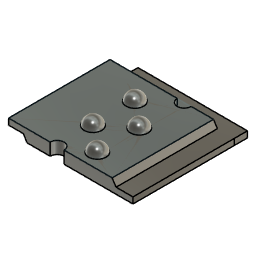
Rivets-Double riveted zig-zag lap joint (Autodesk Fusion 360 design; units mm, degrees)
Autodesk Fusion 360 part; units mm, degrees
sketch "Sketch1" plane through (0, 0, 0) normal (0, 1, 0) x (1, 0, 0)
  line L0 (0, 0) -> (-29, 0)
  line L1 (0, 0) -> (29, 0)
  line L2 (29, 0) -> (29, -7)
  line L3 (29, 0) -> (29, 7)
  line L4 (-29, 0) -> (-29, -7)
  line L5 (-29, 0) -> (-29, 7)
  line L6 (29, 0) -> (53, 0)
  line L7 (-29, 0) -> (-53, 0)
  line L8 (-29, -7) -> (-70, -7)
  line L9 (-70, -7) -> (48.4788, -7)
  line L10 (-29, 7) -> (72.2751, 7)
  line L11 (53, 0) -> (48.4788, -7)
  line L12 (-53, 0) -> (-70, 0)
  line L13 (53, 0) -> (72.2751, 0)
  line L14 (72.2751, 0) -> (72.2751, 7)
  line L15 (-29, -7) -> (-53, -7)
  line L16 (-53, 0) -> (-49.003, 7)
  line L17 (0, 7) -> (-49.003, 7)
  line L18 (-70, -7) -> (-70, 0)
  dimension "d1" = 29
  dimension "d2" = 29
  dimension "d3" = 7
  dimension "d4" = 7
  dimension "d5" = 7
  dimension "d6" = 7
  dimension "d8" = 24
  dimension "d9" = 24
  dimension "d15" = 24
  dimension "d16" = 7
  constraint coincident L0.start L1.start
  constraint horizontal L0
  constraint parallel L0 L1
  constraint perpendicular L1 L2
  constraint perpendicular L1 L3
  constraint perpendicular L0 L4
  constraint perpendicular L0 L5
  constraint perpendicular L2 L6
  constraint perpendicular L5 L7
  constraint perpendicular L4 L8
  constraint perpendicular L2 L9
  constraint perpendicular L3 L10
  constraint parallel L7 L12
  constraint parallel L10 L13
  constraint perpendicular L10 L14
  constraint perpendicular L4 L15
  constraint coincident L10 L17.start
  constraint perpendicular L5 L17
  constraint perpendicular L12 L18
  measures "d1" distance of L0.start L0.end
  measures "d2" distance of L0.start L1.end
  measures "d3" distance of L1.end L2.end
  measures "d4" distance of L1.end L3.end
  measures "d5" distance of L0.end L4.end
  measures "d6" distance of L0.end L5.end
  measures "d8" distance of L1.end L6.end
  measures "d9" distance of L0.end L7.end
  measures "d15" distance of L4.end L15.end
  measures "d16" distance of L15.end L7.end
extrude "Extrude1" add sketch "Sketch1" along normal blind 86 makes body 1
sketch "Sketch2" plane through (0, 0, 0) normal (0, 1, 0) x (1, 0, 0)
ref_plane "WorkPlane1" through (-14.5, 0, 7) normal (0, 0, 1) x (1, 0, 0)
sketch "Sketch3" plane through (0, 0, 7) normal (0, 0, 1) x (1, 0, 0)
  line L0 (0, 0) -> (14.5, 0)
  line L1 (0, 0) -> (-14.5, 0)
  circle A0 centre (14.5, 17) radius 8
  circle A1 centre (14.5, 65) radius 8
  circle A2 centre (-14.5, 41) radius 8
  arc A3 (-6.5, 0) -> (-22.5, 0) centre (-14.5, 0) ccw
  line L2 (-22.5, 0) -> (-14.5, 0)
  dimension "d25" = 14.5
  dimension "d26" = 14.5
  dimension "d29" = 16
  dimension "d31" = 16
  dimension "d32" = 48
  dimension "d33" = 16
  dimension "d35" = 16
  constraint coincident L0.start L1.start
  constraint horizontal L0
  constraint parallel L0 L1
  constraint coincident L1.end A3.centre
  constraint parallel L0 L2
  constraint coincident L1 A3.start
  measures "d25" distance of L0.start L0.end
  measures "d26" distance of L0.start L1.end
  measures "d29" diameter of A3
  measures "d31" diameter of A0
  measures "d32" distance of A0.centre A1.centre
  measures "d33" diameter of A1
  measures "d35" diameter of A2
sketch "Sketch4" plane through (0, 0, 0) normal (0, 1, 0) x (1, 0, 0)
sketch "Sketch5" plane through (0, 86, 0) normal (0, 1, 0) x (-1, 0, 0)
  line L0 (70, 7) -> (-48.4788, 7)
  line L1 (-48.4788, 7) -> (-53, 0)
  line L2 (-53, 0) -> (-72.2751, 0)
  line L3 (-72.2751, 0) -> (-72.2751, -7)
  line L4 (-72.2751, -7) -> (49.003, -7)
  line L5 (49.003, -7) -> (53, 0)
  line L6 (53, 0) -> (70, 0)
  line L7 (70, 0) -> (70, 7)
  line L8 (-72.2751, 0) -> (-72.2751, -7)
  line L9 (-72.2751, -7) -> (49.003, -7)
  line L10 (53, 0) -> (70, 0)
  line L11 (70, 7) -> (-48.4788, 7)
  line L12 (-53, 0) -> (-72.2751, 0)
  constraint coincident L2.end L3.start
  constraint coincident L3.end L4.start
  constraint coincident L4.end L5.start
  constraint coincident L5.end L6.start
  constraint coincident L6.end L7.start
  constraint coincident L0.start L7.end
  constraint coincident L0.end L1.start
  constraint coincident L1.end L2.start
extrude "Extrude2" add sketch "Sketch5" along normal blind 30 bodies 1
sketch "Sketch6" plane through (0, 0, 7) normal (0, 0, 1) x (-1, 0, 0)
  line L0 (70, 0) -> (-48.4788, 0)
  line L1 (-48.4788, 0) -> (-48.4788, -116)
  line L2 (-48.4788, -116) -> (70, -116)
  line L3 (70, -116) -> (70, 0)
  circle A0 centre (14.5, -89) radius 8
  dimension "d40" = 16
  measures "d40" diameter of A0
sketch "Sketch7" plane through (0, 0, 7) normal (0, 0, 1) x (-1, 0, 0)
extrude "Extrude3" cut sketch "Sketch6" sketch "Sketch3" against normal blind 14 contours A0 of sketch 2 bodies 1
sketch "Sketch8" plane through (0, 0, 0) normal (0, 1, 0) x (1, 0, 0)
  line L0 (-129, 0) -> (-129, -7)
  line L1 (-129, -7) -> (-121, -7)
  line L2 (-121, -7) -> (-121, 0)
  line L3 (-129, -7) -> (-119, -7)
  line L4 (-129, -7) -> (-129, -17)
  arc A0 (-129, -17) -> (-119, -7) centre (-129, -7) ccw
  arc A1 (-119, 7) -> (-129, 17) centre (-129, 7) ccw
  line L5 (-129, 7) -> (-129, 17)
  line L6 (-129, 7) -> (-119, 7)
  line L7 (-121, 7) -> (-121, 0)
  line L8 (-129, 0) -> (-129, 7)
  dimension "d45" = 7
  dimension "d46" = 8
  dimension "d47" = 7
  dimension "d50" = 10
  dimension "d51" = 10
  constraint vertical L0
  constraint perpendicular L0 L1
  constraint perpendicular L1 L2
  constraint perpendicular L2 L3
  constraint perpendicular L1 L4
  measures "d45" distance of L0.start L0.end
  measures "d46" distance of L0.end L1.end
  measures "d47" distance of L1.end L2.end
  measures "d50" distance of L0.end L3.end
  measures "d51" distance of L0.end L4.end
sketch "Sketch9" plane through (0, 0, 0) normal (0, 1, 0) x (1, 0, 0)
  line L0 (-129, -17) -> (-129, 17)
  constraint vertical L0
revolve "Revolve1" add sketch "Sketch8" angle 360 about axis through (-129, 0, 17) along (0, 0, -1) separate body makes body 2
copy_body "CopyPasteBodies1" bodies 2 makes body 3
move_body "Move1" bodies 3 to x (1, 0, 0) y (0, 1, 0) z (0, 0, 1) at (143.5, 17, 0)
copy_body "CopyPasteBodies2" bodies 2 makes body 4
move_body "Move2" bodies 4 to x (1, 0, 0) y (0, 1, 0) z (0, 0, 1) at (114.5, 41, 0)
copy_body "CopyPasteBodies3" bodies 2 makes body 5
move_body "Move3" bodies 5 to x (1, 0, 0) y (0, 1, 0) z (0, 0, 1) at (114.5, 89, 0)
move_body "Move4" bodies 2 to x (1, 0, 0) y (0, 1, 0) z (0, 0, 1) at (143.5, 65, 0)
sketch "Sketch10" plane through (0, 116, 0) normal (0, 1, 0) x (-1, 0, 0)
sketch "Sketch11" plane through (0, 116, 0) normal (0, 1, 0) x (-1, 0, 0)
  line L0 (-53, 0) -> (-72.2747, 0)
  line L1 (-72.2747, 0) -> (-72.2747, -7)
  line L2 (-72.2747, -7) -> (49, -7)
  line L3 (49, -7) -> (53, 0)
  line L4 (53, 0) -> (-53, 0)
  constraint horizontal L0
  constraint perpendicular L0 L1
  constraint perpendicular L1 L2
  constraint parallel L0 L4
extrude "Extrude4" add sketch "Sketch11" along normal blind 15 bodies 1
sketch "Sketch12" plane through (0, 0, 7) normal (0, 0, 1) x (-1, 0, 0)
  arc A0 (6.5, 0) -> (22.5, 0) centre (14.5, 0) ccw
  line L0 (6.5, 0) -> (-48.4788, 0)
  line L1 (-48.4788, 0) -> (-48.4788, -116)
  line L2 (-48.4788, -116) -> (70, -116)
  line L3 (70, -116) -> (70, 0)
  line L4 (70, 0) -> (22.5, 0)
  circle A1 centre (-14.5, -65) radius 8
  circle A2 centre (14.5, -89) radius 8
  circle A3 centre (-14.5, -17) radius 8
  circle A4 centre (14.5, -41) radius 8
ref_plane "WorkPlane2" through (48.4788, 116, 7) normal (0, 0, 1) x (1, 0, 0)
sketch "Sketch13" plane through (0, 0, 7) normal (0, 0, 1) x (1, 0, 0)
  circle A0 centre (15, 116) radius 8
  dimension "d56" = 16
  measures "d56" diameter of A0
extrude "Extrude5" cut sketch "Sketch13" against normal blind 7 bodies 1
